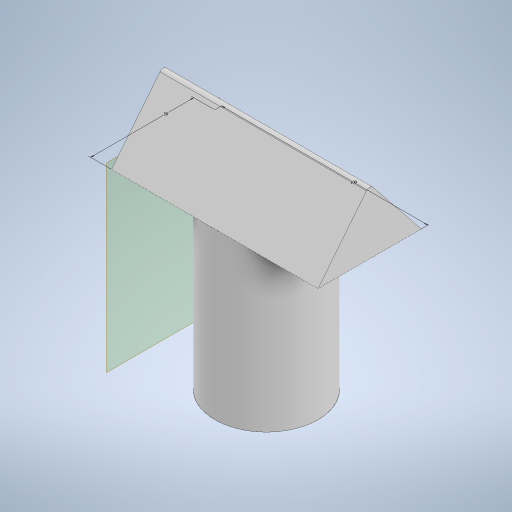
# Autodesk Inventor part: rotator_flat
Saved by Autodesk Inventor 2023.1 (Build 271208000, 208)
## iProperties
Created: 2022-10-07
Part Number: rotator_flat
Material: Generic
Document SubType Name: Modeling
Designer: swang
Density: 1 g/cm^3
Appearance: Default
Author: swang
## iProperties of the stored document rotator_round_3DPrint.ipt
Created: 2022-10-07
Part Number: rotator_round_3DPrint
Material: Generic
Document SubType Name: Modeling
Designer: swang
Density: 1 g/cm^3
Appearance: Default
Author: swang
Autodesk Inventor part; units mm, degrees
ref_plane "YZ Plane" through (0, 0, 0) normal (1, 0, 0) x (0, 1, 0)
ref_plane "XZ Plane" through (0, 0, 0) normal (0, 1, 0) x (-1, 0, 0)
ref_plane "XY Plane" through (0, 0, 0) normal (0, 0, 1) x (1, 0, 0)
sketch "Sketch1" plane through (0, 0, 0) normal (0, 1, 0) x (-1, 0, 0)
  circle A0 centre (0, 0) radius 25
  dimension "d0" = 50
  constraints: 1 centre point, 1 coincident
  measures "d0" diameter of A0
extrude "Extrusion1" add sketch "Sketch1" along normal blind 80
sketch "Sketch3" plane through (0, 80, 0) normal (0, 1, 0) x (1, 0, 0)
  line L0 (-50, -25) -> (50, -25) construction
  line L1 (50, -25) -> (50, 25) construction
  line L2 (50, 25) -> (-50, 25) construction
  line L3 (-50, 25) -> (-50, -25) construction
  line L4 (-50, -25) -> (50, 25) construction
  line L5 (50, -25) -> (-50, 25) construction
  point P0 (0, 0)
  dimension "d7" = 100
  dimension "d8" = 50
  constraints: 12 end point, 2 midpoint, 2 parallel, 1 horizontal, 1 perpendicular
  measures "d7" distance of L1.end L2.end
  measures "d8" distance of L2.end L0.start
ref_plane "Work Plane2" through (-50, 80, -25) normal (-1, 0, 0) x (0, 0, 1)
sketch "Sketch5" plane through (-50, 80, -25) normal (-1, 0, 0) x (0, 0, 1)
  line L0 (50, 0) -> (0, 0)
  line L1 (0, 0) -> (23.4393, 29.2507)
  line L2 (26.5607, 29.2507) -> (50, 0)
  line L3 (50, 0) -> (0, 0) projected
  line L4 (25, 0) -> (25, 74.1504)
  arc A0 (26.5607, 29.2507) -> (23.4393, 29.2507) centre (25, 28) ccw
  point P0 (25, -80)
  point P1 (25, 31.1983)
  point P2 (25, 30)
  dimension "d13" = 2
  dimension "d14" = 30
  constraints: 8 end point, 3 point on circle, 3 point on line, 2 tangent, 1 centre point, 1 horizontal, 1 midpoint, 1 vertical
  measures "d13" radius of A0
  measures "d14" distance from line of L0 point (25, 30)
extrude "Extrusion3" add sketch "Sketch5" against normal blind 100
body "Solid1"
